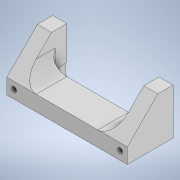
# Autodesk Inventor part: 3DPrintedPrintHeadRetainingFrame_FDM
Saved by Autodesk Inventor 2021 (Build 250183000, 183)
## iProperties
Created: 2021-10-26
Part Number: 3DPrintedPrintHeadRetainingFrame_FDM
Material: Generic
Document SubType Name: Sheet Metal
Designer: Unit-005
Density: 1 g/cm^3
Sheet Metal Rule: Default
Appearance: Default
Author: Unit-005
## iProperties of the stored document _3DPrint.ipt
Created: 2021-10-26
Part Number: _3DPrint
Material: Generic
Document SubType Name: Modeling
Designer: Unit-005
Density: 1 g/cm^3
Appearance: Default
Author: Unit-005
Autodesk Inventor part; units mm, degrees
ref_plane "YZ Plane" through (0, 0, 0) normal (1, 0, 0) x (0, 1, 0)
ref_plane "XZ Plane" through (0, 0, 0) normal (0, 1, 0) x (-1, 0, 0)
ref_plane "XY Plane" through (0, 0, 0) normal (0, 0, 1) x (1, 0, 0)
sketch "Sketch1" plane through (0, 0, 0) normal (0, 0, 1) x (1, 0, 0)
  line L0 (-50.0126, 6.35) -> (50.0126, 6.35)
  line L1 (50.0126, 6.35) -> (50.0126, -6.35)
  line L2 (50.0126, -6.35) -> (-50.0126, -6.35)
  line L3 (-50.0126, -6.35) -> (-50.0126, 6.35)
  line L4 (-50.0126, 6.35) -> (50.0126, -6.35) construction
  line L5 (50.0126, 6.35) -> (-50.0126, -6.35) construction
  point P0 (0, 0)
  dimension "d0" = 100.0252
  dimension "d1" = 12.7
  constraints: 12 end point, 2 midpoint, 2 parallel, 1 horizontal, 1 perpendicular
  measures "d0" distance of L1.end L2.end
  measures "d1" distance of L0.end L1.end
extrude "Extrusion1" add sketch "Sketch1" along normal blind 25.4
sketch "Sketch2" plane through (0, 0, 0) normal (0, 0, 1) x (1, 0, 0)
  line L0 (-50.0126, -6.35) -> (50.0126, -6.35) projected
  line L1 (-50.0126, 6.35) -> (-50.0126, -6.35) projected
  line L2 (50.0126, 6.35) -> (-50.0126, 6.35) projected
  line L3 (50.0126, -6.35) -> (50.0126, 6.35) projected
  line L4 (-70.0176, 0) -> (70.0176, 0) projected
  line L5 (0, -8.89) -> (0, 8.89) projected
  line L6 (50.0126, -6.35) -> (50.0126, 6.35) projected
  line L7 (-50.0126, -6.35) -> (50.0126, -6.35) projected
  line L8 (50.0126, 6.35) -> (38.3286, 6.35)
  line L9 (38.3286, 6.35) -> (38.3286, -6.35)
  line L10 (38.3286, -6.35) -> (50.0126, -6.35)
  line L11 (50.0126, -6.35) -> (50.0126, 6.35)
  point P0 (0, 0)
  point P1 (38.3286, 6.35)
  point P2 (38.3286, -6.35)
  dimension "d4" = 11.684
  constraints: 8 end point, 2 parallel, 1 horizontal, 1 perpendicular, 1 point on line
  measures "d4" distance of L10.end L9.end
extrude "Extrusion2" add sketch "Sketch2" against normal blind 12.7 contours L9 L4 L3 L0 | L9 L2 L3 L4
mirror "Mirror1" about plane through (0, 0, 0) normal (1, 0, 0) of "Extrusion2"
fillet "Fillet1" radius 3.175 2 edges at (38.3286, 0, 0) (-38.3286, 0, 0)
sketch "Sketch3" plane through (0, 0, 0) normal (0, 0, -1) x (-1, 0, 0)
  line L0 (70.0176, 0) -> (-70.0176, 0) projected
  line L1 (0, -8.89) -> (0, 8.89) projected
  line L2 (35.1536, 6.35) -> (35.1536, -6.35) projected
  line L3 (-35.1536, 6.35) -> (35.1536, 6.35) projected
  line L4 (-35.1536, -6.35) -> (-35.1536, 6.35) projected
  line L5 (35.1536, -6.35) -> (-35.1536, -6.35) projected
  circle A0 centre (0, -4.1402) radius 2.0574
  point P0 (0, 0)
  dimension "d9" = 4.1148
  dimension "d10" = 2.2098
  constraints: 1 centre point, 1 point on line
  measures "d9" diameter of A0
  measures "d10" distance from line of L5 A0.centre
extrude "Extrusion3" cut sketch "Sketch3" against normal blind 1.5875 contours A0 L1 | L1 A0
pattern_linear "Rectangular Pattern1" count 11 spacing 6.35 along (1, 0, 0) of "Extrusion3" first direction both ways yes
sketch "Sketch4" plane through (0, 0, -12.7) normal (0, 0, -1) x (-1, 0, 0)
  line L0 (70.0176, 0) -> (-70.0176, 0) projected
  line L1 (0, -8.89) -> (0, 8.89) projected
  line L2 (-50.0126, -6.35) -> (-38.3286, -6.35) projected
  line L3 (-38.3286, -6.35) -> (-38.3286, 6.35) projected
  line L4 (-38.3286, 6.35) -> (-50.0126, 6.35) projected
  line L5 (-50.0126, 6.35) -> (-50.0126, -6.35) projected
  line L6 (50.0126, -6.35) -> (38.3286, -6.35) projected
  line L7 (50.0126, 6.35) -> (50.0126, -6.35) projected
  line L8 (38.3286, 6.35) -> (50.0126, 6.35) projected
  line L9 (38.3286, -6.35) -> (38.3286, 6.35) projected
  line L10 (-38.3286, -6.35) -> (-38.3286, 6.35) projected
  line L11 (-38.3286, 3.683) -> (-39.3446, 3.683)
  line L12 (-39.3446, 3.683) -> (-39.3446, -5.842)
  line L13 (-39.3446, -5.842) -> (-38.3286, -5.842)
  line L14 (-38.3286, -5.842) -> (-38.3286, 3.683)
  point P0 (0, 0)
  point P1 (-38.3286, 3.683)
  dimension "d19" = 1.016
  dimension "d20" = 9.525
  dimension "d21" = 0.508
  constraints: 8 end point, 2 parallel, 1 horizontal, 1 perpendicular, 1 point on line
  measures "d19" distance of L13.end L12.end
  measures "d20" distance of L12.end L11.end
  measures "d21" distance between parallel lines of L2 L13
extrude "Extrusion4" cut sketch "Sketch4" against normal blind 6.35 contours L3 L13 L12 L0 | L0 L12 L11 L3
mirror "Mirror2" about plane through (0, 0, 0) normal (1, 0, 0) of "Extrusion4"
sketch "Sketch5" plane through (0, 0, -12.7) normal (0, 0, -1) x (-1, 0, 0)
  line L0 (-38.3286, -5.842) -> (-39.3446, -5.842) projected
  line L1 (-39.3446, -5.842) -> (-39.3446, 3.683) projected
  line L2 (-39.3446, 3.683) -> (-38.3286, 3.683) projected
  line L3 (-38.3286, 3.683) -> (-38.3286, 6.35) projected
  line L4 (-38.3286, 6.35) -> (-50.0126, 6.35) projected
  line L5 (-50.0126, 6.35) -> (-50.0126, -6.35) projected
  line L6 (-50.0126, -6.35) -> (-38.3286, -6.35) projected
  line L7 (-38.3286, -6.35) -> (-38.3286, -5.842) projected
  line L8 (47.9806, -6.35) -> (47.9806, 6.35) projected
  line L9 (50.0126, 6.35) -> (50.0126, -6.35) projected
  line L10 (38.3286, 3.683) -> (39.3446, 3.683) projected
  line L11 (39.3446, 3.683) -> (39.3446, -5.842) projected
  line L12 (39.3446, -5.842) -> (38.3286, -5.842) projected
  line L13 (38.3286, -6.35) -> (38.3286, -5.842) projected
  line L14 (50.0126, -6.35) -> (38.3286, -6.35) projected
  line L15 (50.0126, 6.35) -> (50.0126, -6.35) projected
  line L16 (38.3286, 6.35) -> (50.0126, 6.35) projected
  line L17 (38.3286, 3.683) -> (38.3286, 6.35) projected
  line L18 (70.0176, 0) -> (-70.0176, 0) projected
  line L19 (0, -8.89) -> (0, 8.89) projected
  circle A0 centre (-44.0182, 0.6604) radius 3.3782
  point P0 (0, 0)
  dimension "d24" = 6.7564
  dimension "d25" = 7.0104
  dimension "d26" = 5.9944
  constraints: 1 centre point
  measures "d24" diameter of A0
  measures "d25" distance from line of L6 A0.centre
  measures "d26" distance from line of L5 A0.centre
hole "Hole1" at (44.0182, 0.6604, -12.7) direction (0, 0, 1) diameter 4.318 end through all clearance for "Socket Head Cap Screw" size "#8" standard "Ansi Unified Screw Threads"
mirror "Mirror3" about plane through (0, 0, 0) normal (1, 0, 0) of "Hole1"
sketch "Sketch6" plane through (38.3286, 6.35, -12.7) normal (0, 1, 0) x (1, 0, 0)
  line L0 (11.684, -38.1) -> (-88.3412, -38.1) projected
  line L1 (11.684, 0) -> (11.684, -38.1) projected
  line L2 (0, 0) -> (11.684, 0) projected
  line L3 (0, -9.525) -> (0, 0) projected
  arc A0 (-3.175, -12.7) -> (0, -9.525) centre (-3.175, -9.525) ccw projected
  line L4 (-3.175, -12.7) -> (-73.4822, -12.7) projected
  arc A1 (-76.6572, -9.525) -> (-73.4822, -12.7) centre (-73.4822, -9.525) ccw projected
  line L5 (-76.6572, -9.525) -> (-76.6572, 0) projected
  line L6 (-76.6572, 0) -> (-88.3412, 0) projected
  line L7 (-88.3412, 0) -> (-88.3412, -38.1) projected
  line L8 (-108.397, -12.7) -> (31.9938, -12.7) projected
  line L9 (-38.3286, 7.62) -> (-38.3286, -45.72) projected
  line L10 (0, -9.525) -> (0, 0) projected
  line L11 (0, 0) -> (11.684, 0)
  line L12 (11.684, 0) -> (11.684, -38.1)
  line L13 (11.684, -38.1) -> (0, -38.1)
  line L14 (0, -38.1) -> (0, 0)
  line L15 (-88.3412, 0) -> (-88.3412, -38.1)
  line L16 (-76.6572, 0) -> (-88.3412, 0)
  line L17 (-76.6572, -9.525) -> (-76.6572, 0)
  arc A2 (-76.6572, -9.525) -> (-73.4822, -12.7) centre (-73.4822, -9.525) ccw
  line L18 (-76.6572, -9.525) -> (-76.6572, 0)
  line L19 (-76.6572, 0) -> (-88.3412, 0)
  line L20 (-88.3412, 0) -> (-88.3412, -38.1)
  line L21 (-88.3412, -38.1) -> (-76.6572, -38.1)
  line L22 (-76.6572, -38.1) -> (-76.6572, 0)
  point P0 (-38.3286, -12.7)
  constraints: 24 end point, 5 symmetric about line, 2 collinear, 2 parallel, 2 point on circle, 1 centre point, 1 horizontal, 1 perpendicular, 1 other
extrude "Extrusion5" add sketch "Sketch6" along normal blind 25.4 contours L0 L14 L8 L1 | L8 L14 L3 L2 L1 | L0 L7 L8 L22 | L8 L7 L6 L5 L22
chamfer "Chamfer2" distance 25.4 angle 45 2 edges at (-44.1706, 31.75, 25.4) (44.1706, 31.75, 25.4)
fillet "Fillet3" radius 12.7 2 edges at (38.3286, 6.35, 11.1125) (-38.3286, 6.35, 11.1125)
chamfer "Chamfer3" distance 0.254 angle 45 2 edges at (39.3446, 3.683, -9.525) (-39.3446, 3.683, -9.525)
sketch "Sketch7" plane through (-50.0126, -6.35, 25.4) normal (0, -1, 0) x (1, 0, 0)
  line L0 (-20.005, -25.4) -> (120.0302, -25.4) projected
  line L1 (50.0126, -45.72) -> (50.0126, 7.62) projected
  line L2 (14.859, -25.4) -> (85.1662, -25.4) projected
  arc A0 (88.3412, -28.575) -> (85.1662, -25.4) centre (85.1662, -28.575) ccw projected
  line L3 (88.3412, -28.575) -> (88.3412, -38.1) projected
  line L4 (100.0252, -38.1) -> (88.3412, -38.1) projected
  line L5 (100.0252, -38.1) -> (100.0252, 0) projected
  line L6 (0, 0) -> (100.0252, 0) projected
  line L7 (0, 0) -> (0, -38.1) projected
  line L8 (0, -38.1) -> (11.684, -38.1) projected
  line L9 (11.684, -28.575) -> (11.684, -38.1) projected
  arc A1 (14.859, -25.4) -> (11.684, -28.575) centre (14.859, -28.575) ccw projected
  circle A2 centre (50.0126, -20.955) radius 1.5875
  point P0 (50.0126, -25.4)
  dimension "d44" = 3.175
  dimension "d45" = 4.445
  constraints: 1 centre point, 1 point on line
  measures "d44" diameter of A2
  measures "d45" distance from line of L0 A2.centre
extrude "Extrusion6" cut sketch "Sketch7" against normal blind 0.635 contours A2 L1 | L1 A2
pattern_linear "Rectangular Pattern2" count 19 spacing 4.699 along (1, 0, 0) count 5 spacing 4.699 along (0, 0, 1) of "Extrusion6" first direction both ways yes
sketch "Sketch8" plane through (-50.0126, -6.35, 25.4) normal (0, -1, 0) x (1, 0, 0)
  circle A0 centre (92.3036, -2.159) radius 1.5875 projected
  circle A1 centre (87.6046, -2.159) radius 1.5875 projected
  circle A2 centre (82.9056, -2.159) radius 1.5875 projected
  circle A3 centre (78.2066, -2.159) radius 1.5875 projected
  circle A4 centre (73.5076, -2.159) radius 1.5875 projected
  circle A5 centre (68.8086, -2.159) radius 1.5875 projected
  circle A6 centre (64.1096, -2.159) radius 1.5875 projected
  circle A7 centre (59.4106, -2.159) radius 1.5875 projected
  circle A8 centre (54.7116, -2.159) radius 1.5875 projected
  circle A9 centre (50.0126, -2.159) radius 1.5875 projected
  circle A10 centre (45.3136, -2.159) radius 1.5875 projected
  circle A11 centre (40.6146, -2.159) radius 1.5875 projected
  circle A12 centre (35.9156, -2.159) radius 1.5875 projected
  circle A13 centre (31.2166, -2.159) radius 1.5875 projected
  circle A14 centre (26.5176, -2.159) radius 1.5875 projected
  circle A15 centre (21.8186, -2.159) radius 1.5875 projected
  circle A16 centre (17.1196, -2.159) radius 1.5875 projected
  circle A17 centre (12.4206, -2.159) radius 1.5875 projected
  circle A18 centre (7.7216, -2.159) radius 1.5875 projected
  circle A19 centre (92.3036, -6.858) radius 1.5875 projected
  circle A20 centre (87.6046, -6.858) radius 1.5875 projected
  circle A21 centre (82.9056, -6.858) radius 1.5875 projected
  circle A22 centre (78.2066, -6.858) radius 1.5875 projected
  circle A23 centre (73.5076, -6.858) radius 1.5875 projected
  circle A24 centre (68.8086, -6.858) radius 1.5875 projected
  circle A25 centre (64.1096, -6.858) radius 1.5875 projected
  circle A26 centre (59.4106, -6.858) radius 1.5875 projected
  circle A27 centre (54.7116, -6.858) radius 1.5875 projected
  circle A28 centre (50.0126, -6.858) radius 1.5875 projected
  circle A29 centre (45.3136, -6.858) radius 1.5875 projected
  circle A30 centre (40.6146, -6.858) radius 1.5875 projected
  circle A31 centre (35.9156, -6.858) radius 1.5875 projected
  circle A32 centre (31.2166, -6.858) radius 1.5875 projected
  circle A33 centre (26.5176, -6.858) radius 1.5875 projected
  circle A34 centre (21.8186, -6.858) radius 1.5875 projected
  circle A35 centre (17.1196, -6.858) radius 1.5875 projected
  circle A36 centre (12.4206, -6.858) radius 1.5875 projected
  circle A37 centre (7.7216, -6.858) radius 1.5875 projected
  circle A38 centre (92.3036, -11.557) radius 1.5875 projected
  circle A39 centre (87.6046, -11.557) radius 1.5875 projected
  circle A40 centre (82.9056, -11.557) radius 1.5875 projected
  circle A41 centre (78.2066, -11.557) radius 1.5875 projected
  circle A42 centre (73.5076, -11.557) radius 1.5875 projected
  circle A43 centre (68.8086, -11.557) radius 1.5875 projected
  circle A44 centre (64.1096, -11.557) radius 1.5875 projected
  circle A45 centre (59.4106, -11.557) radius 1.5875 projected
  circle A46 centre (54.7116, -11.557) radius 1.5875 projected
  circle A47 centre (50.0126, -11.557) radius 1.5875 projected
  circle A48 centre (45.3136, -11.557) radius 1.5875 projected
  circle A49 centre (40.6146, -11.557) radius 1.5875 projected
  circle A50 centre (35.9156, -11.557) radius 1.5875 projected
  circle A51 centre (31.2166, -11.557) radius 1.5875 projected
  circle A52 centre (26.5176, -11.557) radius 1.5875 projected
  circle A53 centre (21.8186, -11.557) radius 1.5875 projected
  circle A54 centre (17.1196, -11.557) radius 1.5875 projected
  circle A55 centre (12.4206, -11.557) radius 1.5875 projected
  circle A56 centre (7.7216, -11.557) radius 1.5875 projected
  circle A57 centre (92.3036, -16.256) radius 1.5875 projected
  circle A58 centre (87.6046, -16.256) radius 1.5875 projected
  circle A59 centre (82.9056, -16.256) radius 1.5875 projected
  circle A60 centre (78.2066, -16.256) radius 1.5875 projected
  circle A61 centre (73.5076, -16.256) radius 1.5875 projected
  circle A62 centre (68.8086, -16.256) radius 1.5875 projected
  circle A63 centre (64.1096, -16.256) radius 1.5875 projected
  circle A64 centre (59.4106, -16.256) radius 1.5875 projected
  circle A65 centre (54.7116, -16.256) radius 1.5875 projected
  circle A66 centre (50.0126, -16.256) radius 1.5875 projected
  circle A67 centre (45.3136, -16.256) radius 1.5875 projected
  circle A68 centre (40.6146, -16.256) radius 1.5875 projected
  circle A69 centre (35.9156, -16.256) radius 1.5875 projected
  circle A70 centre (31.2166, -16.256) radius 1.5875 projected
  circle A71 centre (26.5176, -16.256) radius 1.5875 projected
  circle A72 centre (21.8186, -16.256) radius 1.5875 projected
  circle A73 centre (17.1196, -16.256) radius 1.5875 projected
  circle A74 centre (12.4206, -16.256) radius 1.5875 projected
  circle A75 centre (7.7216, -16.256) radius 1.5875 projected
  circle A76 centre (92.3036, -20.955) radius 1.5875 projected
  circle A77 centre (87.6046, -20.955) radius 1.5875 projected
  circle A78 centre (82.9056, -20.955) radius 1.5875 projected
  circle A79 centre (78.2066, -20.955) radius 1.5875 projected
  circle A80 centre (73.5076, -20.955) radius 1.5875 projected
  circle A81 centre (68.8086, -20.955) radius 1.5875 projected
  circle A82 centre (64.1096, -20.955) radius 1.5875 projected
  circle A83 centre (59.4106, -20.955) radius 1.5875 projected
  circle A84 centre (54.7116, -20.955) radius 1.5875 projected
  circle A85 centre (45.3136, -20.955) radius 1.5875 projected
  circle A86 centre (40.6146, -20.955) radius 1.5875 projected
  circle A87 centre (35.9156, -20.955) radius 1.5875 projected
  circle A88 centre (31.2166, -20.955) radius 1.5875 projected
  circle A89 centre (26.5176, -20.955) radius 1.5875 projected
  circle A90 centre (21.8186, -20.955) radius 1.5875 projected
  circle A91 centre (17.1196, -20.955) radius 1.5875 projected
  circle A92 centre (12.4206, -20.955) radius 1.5875 projected
  circle A93 centre (7.7216, -20.955) radius 1.5875 projected
  circle A94 centre (50.0126, -20.955) radius 1.5875 projected
  line L0 (14.859, -25.4) -> (85.1662, -25.4) projected
  arc A95 (88.3412, -28.575) -> (85.1662, -25.4) centre (85.1662, -28.575) ccw projected
  line L1 (88.3412, -28.575) -> (88.3412, -38.1) projected
  line L2 (100.0252, -38.1) -> (88.3412, -38.1) projected
  line L3 (100.0252, -38.1) -> (100.0252, 0) projected
  line L4 (0, 0) -> (100.0252, 0) projected
  line L5 (0, 0) -> (0, -38.1) projected
  line L6 (0, -38.1) -> (11.684, -38.1) projected
  line L7 (11.684, -28.575) -> (11.684, -38.1) projected
  arc A96 (14.859, -25.4) -> (11.684, -28.575) centre (14.859, -28.575) ccw projected
  line L8 (-20.005, -25.4) -> (120.0302, -25.4) projected
  line L9 (50.0126, -45.72) -> (50.0126, 7.62) projected
  circle A97 centre (96.2152, -25.4) radius 1.5875
  point P0 (50.0126, -25.4)
  dimension "d54" = 3.175
  dimension "d55" = 3.81
  constraints: 1 centre point, 1 point on line
  measures "d54" diameter of A97
  measures "d55" distance from line of L3 A97.centre
extrude "Extrusion7" cut sketch "Sketch8" against normal blind 1.27 contours A97 L8 | L8 A97
pattern_linear "Rectangular Pattern3" count 3 spacing 3.81 along (0, 0, -1) count 2 spacing 3.81 along (-1, 0, 0) of "Extrusion7"
mirror "Mirror4" about plane through (0, 0, 0) normal (1, 0, 0) of "Extrusion7", "Rectangular Pattern3"
equation "\"d32\" = Thickness"
equation "\"BendRadius\" = Thickness"
equation "\"BendReliefWidth\" = Thickness"
equation "\"BendReliefDepth\" = 0.5 * Thickness"
equation "\"CornerReliefSize\" = 4 * Thickness"
equation "\"MinimumRemnant\" = 2 * Thickness"
equation "\"TransitionRadius\" = BendRadius"
equation "\"JacobiRadiusSize\" = BendRadius"
equation "\"GapSize\" = Thickness"
equation "\"Thickness\" = 3.048"
body "Solid1"
